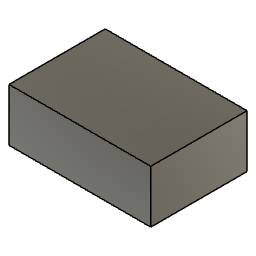
jetson orin 모델 (Autodesk Fusion 360 design; units mm, degrees)
Autodesk Fusion 360 part; units mm, degrees
sketch "스케치1" plane through (0, 0, 0) normal (0, 0, 1) x (1, 0, 0)
  line L0 (70, 47.5) -> (-70, 47.5)
  line L1 (-70, 47.5) -> (-70, -47.5)
  line L2 (-70, -47.5) -> (70, -47.5)
  line L3 (70, -47.5) -> (70, 47.5)
  line L4 (70, 47.5) -> (-70, -47.5) construction
  line L5 (-70, 47.5) -> (70, -47.5) construction
  dimension "d1" = 140
  dimension "d2" = 95
  constraint horizontal L0
  constraint perpendicular L0 L1
  constraint parallel L0 L2
  constraint parallel L1 L3
  constraint coincident L4 origin
  constraint coincident L5 origin
  measures "d1" distance of L1.end L2.end
  measures "d2" distance of L0.end L1.end
extrude "돌출1" add sketch "스케치1" along normal blind 52
